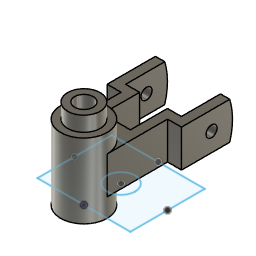
practice_1 v3 (Autodesk Fusion 360 design; units mm, degrees)
Autodesk Fusion 360 part; units mm, degrees
sketch "Sketch1" plane through (0, 0, 0) normal (0, 0, 1) x (1, 0, 0)
  line L0 (-50, 0) -> (50, 0)
  line L1 (50, 0) -> (50, 80)
  line L2 (50, 80) -> (-50, 80)
  line L3 (-50, 80) -> (-50, 0)
  circle A0 centre (0, 40) radius 15
  point P0 (0, 80)
  point P1 (50, 40)
  point P2 (-50, 40)
  point P3 (0, 80)
  point P4 (0, 40)
  dimension "d7" = 30
  constraint horizontal L0
  constraint vertical L1
  constraint horizontal L2
  constraint vertical L3
  constraint midpoint L2 P3
  constraint midpoint L1 P1
  constraint midpoint L3 P2
  constraint coincident P3 P0
  constraint coincident P4 A0.centre
  measures "d7" diameter of A0
extrude "Extrude1" add sketch "Sketch1" along normal blind 15 contours L0 L1 L2 L3 | A0 makes body 1
move_body "Move1" bodies 1 to x (1, 0, 0) y (0, 1, 0) z (0, 0, 1) at (-130, 130, 0)
sketch "Sketch2" plane through (0, 0, 0) normal (0, 0, 1) x (1, 0, 0)
  circle A0 centre (0, 0) radius 40
  circle A1 centre (0, 0) radius 30
  circle A2 centre (0, 0) radius 15
  dimension "d3" = 30
  constraint coincident A0.centre A1.centre
  constraint concentric A1 A2
  measures "d3" diameter of A2
extrude "Extrude2" add sketch "Sketch2" along normal blind 20 separate body contours A0 makes body 2
sketch "Sketch3" plane through (0, 0, 0) normal (0, 0, 1) x (1, 0, 0)
  circle A0 centre (0, 0) radius 15
  dimension "d6" = 30
  constraint coincident A0.centre origin
  measures "d6" diameter of A0
move_body "Move2" bodies 2 to x (1, 0, 0) y (0, 1, 0) z (0, 0, 1) at (0, 0, 60)
move_body "Move3" bodies 1 to x (1, 0, 0) y (0, 1, 0) z (0, 0, 1) at (130, -170, 0)
move_body "Move4" bodies 2 to x (1, 0, 0) y (0, 1, 0) z (0, 0, 1) at (0, 0, -45)
extrude "Extrude3" cut sketch "Sketch3" along normal blind 10 bodies 1
extrude "Extrude4" cut 1 faces at (3.8315, 5.6199, 10) along direction (0, 0, 1) blind 130 on bodies 1 bodies 1
move_body "Move5" bodies 2 1 to x (1, 0, 0) y (0, 1, 0) z (0, 0, 1) at (160, 0, 0)
sketch "Sketch8" plane through (0, 0, 0) normal (0, 1, 0) x (1, 0, 0)
  line L0 (-40, 0) -> (40, 0)
  line L1 (40, 0) -> (40, 100)
  line L2 (40, 100) -> (-40, 100)
  line L3 (-40, 100) -> (-40, 0)
  circle A0 centre (0, 60) radius 16
  dimension "d14" = 32
  dimension "d19" = 40
  constraint horizontal L0
  constraint vertical L1
  constraint horizontal L2
  constraint vertical L3
  measures "d14" diameter of A0
  measures "d19" distance of L2 A0.centre
extrude "Extrude5" add sketch "Sketch8" along normal blind 20 separate body makes body 3
move_body "Move7" bodies 3 to x (1, 0, 0) y (0, 1, 0) z (0, 0, 1) at (0, 0, 20)
fillet "Fillet1" radius 40 1 faces at (13.3333, 6.6667, -80) on bodies 3
copy_body "CopyPasteBodies2" bodies 3 makes body 4
move_body "Move8" bodies 4 to x (1, 0, 0) y (0, 1, 0) z (0, 0, 1) at (0, 100, 0)
move_body "Move9" bodies 1 2 to x (1, 0, 0) y (0, 1, 0) z (0, 0, 1) at (-120, 60, 0)
move_body "Move10" bodies 3 to x (1, 0, 0) y (0, 1, 0) z (0, 0, 1) at (0, 20, -20)
move_body "Move11" bodies 4 to x (1, 0, 0) y (0, 1, 0) z (0, 0, 1) at (0, -20, -20)
move_body "Move12" bodies 3 to x (1, 0, 0) y (0, 1, 0) z (0, 0, 1) at (30, 0, 0)
move_body "Move13" bodies 4 to x (1, 0, 0) y (0, 1, 0) z (0, 0, 1) at (40, 0, 0)
move_body "Move14" bodies 4 to x (0, -1, 0) y (1, 0, 0) z (0, 0, 1) at (-10, 100, 0)
move_body "Move15" bodies 3 to x (0, 1, 0) y (-1, 0, 0) z (0, 0, 1) at (30, 30, 0)
sketch "Sketch10" plane through (0, 0, 0) normal (0, 0, 1) x (1, 0, 0)
  line L0 (0, 0) -> (75, 0)
  line L1 (75, 0) -> (75, 52)
  line L2 (75, 52) -> (0, 52)
  line L3 (0, 52) -> (0, 0)
  dimension "d21" = 75
  dimension "d22" = 52
  dimension "d25" = 75
  dimension "d26" = 52
  constraint horizontal L0
  constraint vertical L1
  constraint horizontal L2
  constraint vertical L3
  constraint coincident L0.start L3.end
  measures "d21" distance of L0.start L0.end
  measures "d22" distance of L0.start L2.end
  measures "d25" distance of L1.end L2.end
  measures "d26" distance of L0.end L1.end
extrude "Extrude6" add sketch "Sketch10" along normal blind 6 separate body makes body 5
sketch "Sketch16" plane through (0, 0, 0) normal (0, -1, 0) x (1, 0, 0)
  line L0 (0, 0) -> (75, 0)
  line L1 (75, 0) -> (75, 6)
  line L2 (75, 6) -> (0, 6)
  line L3 (0, 6) -> (0, 0)
  circle A0 centre (37.5, 46) radius 15
  circle A1 centre (37.5, 46) radius 23
  line L4 (33, 24) -> (42, 24)
  line L5 (42, 24) -> (42, 6)
  line L6 (42, 6) -> (33, 6)
  line L7 (33, 6) -> (33, 24)
  line L8 (0, 46) -> (74, 46)
  point P0 (-2, 3)
  point P1 (0, 3)
  point P2 (75, 3)
  point P3 (37.5, 6)
  point P4 (37.5, 0)
  point P5 (37.5, 46)
  dimension "d28" = 40
  dimension "d29" = 30
  dimension "d30" = 46
  dimension "d31" = 9
  constraint midpoint L3 P1
  constraint midpoint L1 P2
  constraint midpoint L2 P3
  constraint midpoint L0 P4
  constraint coincident P5 A0.centre
  constraint concentric A0 A1
  constraint horizontal L4
  constraint vertical L5
  constraint horizontal L6
  constraint vertical L7
  constraint coincident L2 L5.end
  constraint horizontal L8
  measures "d28" distance of P3 P5
  measures "d29" diameter of A0
  measures "d30" diameter of A1
  measures "d31" distance of L4.start L4.end
extrude "Extrude7" add sketch "Sketch16" against normal blind 52 separate body contours A0 A1 L4 L5 L7 L8 | A0 A1 L8 makes body 6
extrude "Extrude8" add 1 faces at (36, 17.3333, 24) along direction (0, 0, -1) blind 22 on bodies 6 bodies 5 6
extrude "Extrude9" cut sketch "Sketch16" against normal blind 52 contours A0 A1 L8 bodies 5
sketch "Sketch17" plane through (75, 0, 0) normal (1, 0, 0) x (0, 1, 0)
  line L0 (0, 0) -> (52, 0)
  line L1 (52, 0) -> (52, 6)
  line L2 (52, 6) -> (0, 6)
  line L3 (0, 6) -> (0, 0)
  line L4 (22, 3) -> (31, 3)
  line L5 (31, 3) -> (31, 46)
  line L6 (31, 46) -> (22, 46)
  line L7 (22, 46) -> (22, 3)
  point P0 (0, 3)
  point P1 (52, 3)
  point P2 (26, 6)
  point P3 (26, 0)
  point P4 (26, 3)
  constraint midpoint L3 P0
  constraint midpoint L1 P1
  constraint midpoint L2 P2
  constraint midpoint L0 P3
  constraint horizontal L4
  constraint vertical L5
  constraint horizontal L6
  constraint vertical L7
extrude "Extrude10" add sketch "Sketch17" against normal blind 33 contours L2 L5 L6 L7 bodies 5
extrude "Extrude11" cut sketch "Sketch16" against normal blind 52 contours A0 L8 picked at (38.5568, 40.3801) bodies 5
ref_plane "WorkPlane1" through (37.5, 26, 3) normal (-1, 0, 0) x (0, -1, 0)
mirror "Mirror1" about plane through (37.5, 26, 3) normal (-1, 0, 0) of "Extrude10", "Extrude11"
sketch "Sketch18" plane through (0, 0, 0) normal (0, 0, 1) x (1, 0, 0)
  circle A0 centre (0, 0) radius 25
  circle A1 centre (0, 0) radius 17.5
  circle A2 centre (0, 0) radius 10
  dimension "d44" = 50
  dimension "d45" = 35
  dimension "d46" = 20
  constraint coincident A0.centre A1.centre
  constraint concentric A0 A1
  constraint concentric A0 A2
  measures "d44" diameter of A0
  measures "d45" diameter of A1
  measures "d46" diameter of A2
extrude "Extrude12" add sketch "Sketch18" along normal blind 80 separate body contours A0 makes body 7
extrude "Extrude13" add sketch "Sketch18" along normal blind 96 contours A1 bodies 7
sketch "Sketch19" plane through (0, 0, 0) normal (0, 0, 1) x (1, 0, 0)
  line L0 (25, 0) -> (-25, 0)
  line L1 (-25, 0) -> (-25, 35)
  line L2 (-25, 35) -> (25, 35)
  line L3 (25, 35) -> (25, 0)
  dimension "d55" = 35
  constraint horizontal L0
  constraint vertical L1
  constraint horizontal L2
  constraint vertical L3
  measures "d55" distance of L0.end L1.end
extrude "Extrude14" add sketch "Sketch19" along normal blind 60 and the other way blind -20 bodies 7
sketch "Sketch20" plane through (0, 0, 60) normal (0, 0, 1) x (-1, 0, 0)
  arc A0 (-25, 0) -> (25, 0) centre (0, 0) ccw
  line L0 (-25, 0) -> (-25, -35)
  line L1 (-25, -35) -> (25, -35)
  line L2 (25, -35) -> (25, 0)
  line L3 (-15, -65) -> (-25, -65)
  line L4 (-25, -65) -> (-25, -35)
  line L5 (-25, -35) -> (-15, -35)
  line L6 (-15, -35) -> (-15, -65)
  line L7 (15, -35) -> (25, -35)
  line L8 (-15, -65) -> (-40, -65)
  line L9 (-40, -65) -> (-40, -74.8786)
  line L10 (-40, -74.8786) -> (-15, -74.8786)
  line L11 (-15, -74.8786) -> (-15, -65)
  line L12 (-40, -74.8786) -> (-30, -74.8786)
  line L13 (-30, -74.8786) -> (-30, -119.8786)
  line L14 (-30, -119.8786) -> (-40, -119.8786)
  line L15 (-40, -119.8786) -> (-40, -74.8786)
  point P0 (-15, -35)
  point P1 (15, -35)
  point P2 (25, -65)
  point P3 (25, 0)
  point P4 (-24.9893, -65.0273)
  point P5 (-15, -65)
  point P6 (15, -65)
  point P7 (-49.9889, -64.8786)
  point P8 (-50, -74.8786)
  dimension "d57" = 25
  dimension "d58" = 10
  dimension "d59" = 25
  dimension "d60" = 10
  dimension "d61" = 45
  constraint coincident L1 P0
  constraint coincident L1 P1
  constraint coincident P3 A0.end
  constraint horizontal L3
  constraint vertical L4
  constraint horizontal L5
  constraint vertical L6
  constraint coincident L0.end L1.start
  constraint coincident P5 L3.start
  constraint horizontal L7
  constraint coincident P1 L7.start
  constraint horizontal L8
  constraint vertical L9
  constraint horizontal L10
  constraint vertical L11
  constraint horizontal L12
  constraint vertical L13
  constraint horizontal L14
  constraint vertical L15
  measures "d57" distance of P4 P7
  measures "d58" vertical distance of P7 P8
  measures "d59" distance of P5 L8.end
  measures "d60" distance of L9.end L12.end
  measures "d61" distance of L9.end L14.end
extrude "Extrude15" add sketch "Sketch20" against normal blind 40 contours L1 L3 L4 L5 L6 L8 bodies 7
extrude "Extrude16" add sketch "Sketch20" against normal blind 40 contours L3 L8 L9 L10 L11 L12 bodies 7
extrude "Extrude17" add sketch "Sketch20" against normal blind 40 contours L10 L12 L13 L14 L15 bodies 7
sketch "Sketch21" plane through (30, 0, 0) normal (-1, 0, 0) x (0, -1, 0)
  line L0 (-74.8786, 60) -> (-119.8786, 60)
  line L1 (-119.8786, 60) -> (-119.8786, 20)
  line L2 (-119.8786, 20) -> (-74.8786, 20)
  line L3 (-74.8786, 20) -> (-74.8786, 60)
  circle A0 centre (-97.3786, 40) radius 6
  point P0 (-119.8786, 40)
  point P1 (-74.8786, 40)
  point P2 (-97.3786, 60)
  point P3 (-97.3786, 20)
  point P4 (-97.3786, 40)
  dimension "d68" = 12
  constraint midpoint L1 P0
  constraint midpoint L3 P1
  constraint midpoint L0 P2
  constraint midpoint L2 P3
  constraint coincident P4 A0.centre
  measures "d68" diameter of A0
extrude "Extrude18" cut sketch "Sketch21" against normal blind 54 contours A0 bodies 7
ref_plane "WorkPlane2" through (0, 17.5, 40) normal (-1, 0, 0) x (0, -1, 0)
mirror "Mirror2" about plane through (0, 17.5, 40) normal (-1, 0, 0) of "Extrude15", "Extrude16", "Extrude17", "Extrude18"
sketch "Sketch22" plane through (-40, 0, 0) normal (-1, 0, 0) x (0, -1, 0)
  circle A0 centre (-97.3786, 40) radius 6
  line L0 (-65, 60) -> (-119.8786, 60)
  line L1 (-119.8786, 60) -> (-119.8786, 20)
  line L2 (-119.8786, 20) -> (-65, 20)
  line L3 (-65, 20) -> (-65, 60)
  line L4 (-119.8786, 40) -> (-49.8786, 40) construction
  circle A1 centre (-49.8786, 40) radius 70
  dimension "d73" = 70
  constraint midpoint L1 L4.start
  constraint perpendicular L1 L4
  constraint coincident L4.end A1.centre
  constraint coincident L4.start A1
  measures "d73" distance of L4.start L4.end
extrude "Extrude19" cut sketch "Sketch22" against normal blind 205 contours L0 L1 A1 | L1 L2 A1 bodies 7
hidden bodies 1 2 3 4 5
